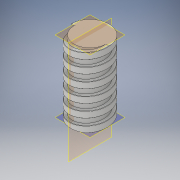
# Autodesk Inventor part: macho_custom
Saved by Autodesk Inventor 2019 (Build 230136000, 136)
## iProperties
Created: 2018-12-23
Part Number: macho_custom
Material: Generic
Document SubType Name: Modeling
Designer: assman
Density: 1 g/cm^3
Appearance: Default
Author: assman
Autodesk Inventor part; units mm, degrees
ref_plane "XZ Plane" through (0, 0, 0) normal (0, 1, 0) x (-1, 0, 0)
ref_plane "XY Plane" through (0, 0, 0) normal (0, 0, 1) x (1, 0, 0)
sketch "Sketch1" plane through (0, 0, 0) normal (0, 1, 0) x (-1, 0, 0)
  circle A0 centre (0, 0) radius 10
  dimension "d0" = 20
  constraints: 1 centre point, 1 coincident
  measures "d0" diameter of A0
extrude "Extrusion1" add sketch "Sketch1" along normal blind 50
sketch "Sketch3" plane through (0, 0, 0) normal (1, 0, 0) x (0, 1, 0)
  line L0 (50, -10) -> (50, 10) construction
  line L1 (0, 10) -> (0, -10) construction
  line L2 (-4.9107, 0) -> (65.9524, 0) construction
  line L3 (0, -10) -> (0, -12)
  line L4 (0, -12) -> (3, -12)
  line L5 (3, -12) -> (4.0057, -12)
  line L6 (4.0057, -12) -> (4.0057, -10)
  line L7 (4.0057, -10) -> (0, -10)
  point P0 (0, 0)
  dimension "d3" = 2
  dimension "d4" = 3
  constraints: 12 end point, 2 perpendicular, 1 horizontal, 1 parallel, 1 point on line, 1 vertical
  measures "d3" distance of L1.end L3.end
  measures "d4" distance of L3.end L4.end
coil "Coil1" sketch "Sketch3" operation add axis through (0, -4.9107, 0) along (0, 1, 0) pitch 8 turns 7 hand right
ref_plane "Work Plane1" through (0, 5, 0) normal (0, -1, 0) x (1, 0, 0)
split "Split1" plane through (0, 5, 0) removes the side toward (0, -1, 0)
ref_plane "Work Plane2" through (0, 50, 0) normal (0, 1, 0) x (1, 0, 0)
split "Split2" plane through (0, 50, 0) removes the side toward (0, 1, 0)
fillet "Fillet1" radius 0.2 12 edges at (-11.0968, 6.5029, 4.5673) (12, 10.0057, 0) (-12, 14.0057, 0) (-12, 22.0057, 0) (12, 18.0057, 0) (-12, 30.0057, 0) (12, 26.0057, 0) (-12, 38.0057, 0) (12, 34.0057, 0) (-12, 46.0057, 0) (12, 42.0057, 0) (8.4662, 49.0029, 8.5043)
fillet "Fillet2" radius 0.2 12 edges at (-12, 10, 0) (12, 14, 0) (-12, 18, 0) (11.0866, 6.5, -4.5922) (12, 22, 0) (-12, 26, 0) (12, 30, 0) (-12, 34, 0) (12, 38, 0) (-12, 42, 0) (12, 46, 0) (-8.4853, 49, -8.4853)
body "Solid1"
